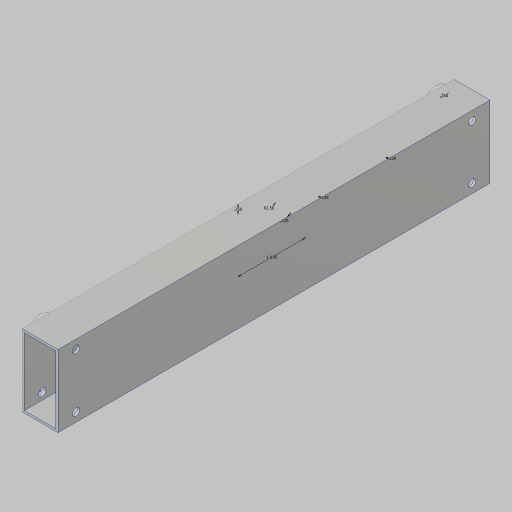
# Autodesk Inventor part: CL7-015
Saved by Autodesk Inventor 2023.5 (Build 275446000, 446)
## iProperties
RuleStatus: InUse
Created: 2025-03-19
Part Number: CL7-015
Material: Aluminum 6061
Document SubType Name: Modeling
Designer: slick
Mass: 304.185 g
Surface Area: 718.547 cm^2
Volume: 112.661 cm^3
Density: 2.7 g/cm^3
Appearance: Aluminum - Flat
AfterDocNew0: SHOW
AfterDocOpen0: SHOW
Author: slick
Autodesk Inventor part; units mm, degrees
ref_plane "YZ Plane" through (0, 0, 0) normal (1, 0, 0) x (0, 1, 0)
ref_plane "XZ Plane" through (0, 0, 0) normal (0, 1, 0) x (-1, 0, 0)
ref_plane "XY Plane" through (0, 0, 0) normal (0, 0, 1) x (1, 0, 0)
sketch "Sketch1" plane through (0, 0, 0) normal (0, 0, 1) x (1, 0, 0)
  line L0 (-12.7, -25.4) -> (12.7, -25.4)
  line L1 (12.7, -25.4) -> (12.7, 25.4)
  line L2 (12.7, 25.4) -> (-12.7, 25.4)
  line L3 (-12.7, 25.4) -> (-12.7, -25.4)
  line L4 (-12.7, -25.4) -> (12.7, 25.4) construction
  line L5 (12.7, -25.4) -> (-12.7, 25.4) construction
  line L6 (-11.1125, 23.8125) -> (11.1125, 23.8125)
  line L7 (11.1125, 23.8125) -> (11.1125, -23.8125)
  line L8 (11.1125, -23.8125) -> (-11.1125, -23.8125)
  line L9 (-11.1125, -23.8125) -> (-11.1125, 23.8125)
  point P0 (0, 0)
  dimension "width" = 25.4
  dimension "height" = 50.8
  dimension "thickness" = 1.5875
  constraints: 20 end point, 4 parallel, 2 midpoint, 2 perpendicular, 1 horizontal, 3 other
  measures "width" distance of L2.end L1.end
  measures "height" distance of L1.end L0.end
  measures "thickness" distance between parallel lines of L2 L6
extrude "Extrusion1" add sketch "Sketch1" along normal mid plane 304.8
sketch "Sketch2" plane through (-12.7, -25.4, 152.4) normal (-1, 0, 0) x (0, 0, 1)
  line L0 (-292.1, 44.45) -> (-292.1, 6.35) construction
  line L1 (-304.8, 0) -> (-304.8, 50.8) construction
  line L2 (0, 50.8) -> (0, 0) construction
  point P0 (-152.4, 25.4)
  point P1 (-12.7, 6.35)
  point P2 (-12.7, 44.45)
  point P3 (-292.1, 25.4)
  dimension "d5" = 12.7
  dimension "d6" = 12.7
  dimension "d7" = 38.1
  constraints: 3 horizontal alignment, 2 end point, 2 vertical alignment, 1 midpoint, 1 vertical
  measures "d5" distance between parallel lines of L1 L0
  measures "d6" distance from line of L2 point (-12.7, 44.45)
  measures "d7" distance of L0.start L0.end
hole "Hole1" at (-12.7, 19.05, -139.7) at (-12.7, -19.05, -139.7) at (-12.7, -19.05, 139.7) at (-12.7, 19.05, 139.7) direction (1, 0, 0) diameter 5.1054 end through all clearance for "Flat Head Machine Screw (82)" size "#10" standard "Ansi Unified Screw Threads"
sketch "Sketch3" plane through (-12.7, -25.4, 152.4) normal (-1, 0, 0) x (0, 0, 1)
  circle A0 centre (-12.7, 6.35) radius 2.5527 construction
  circle A1 centre (-292.1, 44.45) radius 2.5527 construction
  circle A2 centre (-292.1, 6.35) radius 2.5527 construction
  circle A3 centre (-12.7, 44.45) radius 2.5527 construction
  line L0 (0, 0) -> (-304.8, 0) construction
  line L1 (0, 50.8) -> (0, 0) construction
  line L2 (-304.8, 50.8) -> (0, 50.8) construction
  line L3 (-304.8, 0) -> (-304.8, 50.8) construction
  line L4 (-6.35, 44.45) -> (-6.35, 6.35) construction
  line L5 (-6.35, 6.35) -> (-298.45, 6.35) construction
  line L6 (-298.45, 6.35) -> (-298.45, 44.45) construction
  line L7 (-298.45, 44.45) -> (-6.35, 44.45) construction
  circle A4 centre (-292.1, 44.45) radius 8.9027 construction
  circle A5 centre (-292.1, 6.35) radius 2.5527 construction
  circle A6 centre (-292.1, 6.35) radius 8.9027 construction
  circle A7 centre (-12.7, 6.35) radius 8.9027 construction
  circle A8 centre (-12.7, 44.45) radius 2.5527 construction
  circle A9 centre (-12.7, 44.45) radius 8.9027 construction
  line L8 (-152.4, 44.45) -> (-152.4, 6.35) construction
  line L9 (-152.4, 6.35) -> (-175.5196, 44.45) construction
  line L10 (-175.5196, 44.45) -> (-198.6393, 6.35) construction
  line L11 (-200.025, 6.35) -> (-223.1446, 44.45) construction
  line L12 (-223.1446, 44.45) -> (-246.2643, 6.35) construction
  line L13 (-247.65, 6.35) -> (-270.7696, 44.45) construction
  line L14 (-270.7696, 44.45) -> (-293.8893, 6.35) construction
  line L15 (-201.3536, 7.9971) -> (-175.5196, 50.5702) construction
  line L16 (-175.5196, 50.5702) -> (-155.575, 17.7024) construction
  line L17 (-155.575, 17.7024) -> (-155.575, 44.45) construction
  line L18 (-197.3107, 7.9971) -> (-223.1446, 50.5702) construction
  line L19 (-223.1446, 50.5702) -> (-248.9786, 7.9971) construction
  line L20 (-244.9357, 7.9971) -> (-270.7696, 50.5702) construction
  line L21 (-270.7696, 50.5702) -> (-296.6036, 7.9971) construction
  point P0 (-152.4, 25.4)
  dimension "d15" = 6.35
  dimension "d16" = 6.35
  dimension "d19" = 62.5
  dimension "d22" = 47.625
  dimension "d27" = 3.175
  dimension "d28" = 3.175
  dimension "d29" = 3.175
  constraints: 36 end point, 4 centre point, 3 coincident, 3 equal radius, 2 midpoint, 2 point on line, 1 equal length, 1 horizontal, 17 other
  measures "d15" distance between parallel lines of L2 L7
  measures "d16" radial gap between concentric circles of A1 A4
  measures "d19" angle of L9 L10
  measures "d22" distance of L8.end L11.start
  measures "d27" distance between parallel lines of L10 L15
  measures "d28" distance between parallel lines of L11 L18
  measures "d29" distance between parallel lines of L13 L20
body "Solid1"
